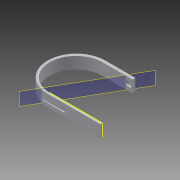
# Autodesk Inventor part: PinewoodFinish
Saved by Autodesk Inventor 2013 (Build 170138000, 138)
## iProperties
Created: 2015-05-15
Part Number: PinewoodFinish
Material: Generic
Document SubType Name: Modeling
Designer: joshgunnar
Density: 1 g/cm^3
Author: joshgunnar
Autodesk Inventor part; units mm, degrees
ref_plane "YZ Plane" through (0, 0, 0) normal (1, 0, 0) x (0, 1, 0)
ref_plane "XZ Plane" through (0, 0, 0) normal (0, 1, 0) x (-1, 0, 0)
sketch "Sketch1" plane through (0, 0, 0) normal (0, 0, 1) x (1, 0, 0)
  line L0 (0, 0) -> (88.9, 0)
  line L1 (88.9, 0) -> (88.9, 3.5)
  line L2 (88.9, 3.5) -> (0, 3.5)
  line L3 (0, 3.5) -> (0, 0)
  line L4 (0, 92.4) -> (50.8, 92.4)
  line L5 (50.8, 92.4) -> (50.8, 97.4)
  line L6 (50.8, 97.4) -> (0, 97.4)
  line L7 (0, 97.4) -> (0, 92.4)
  arc A0 (0, 92.4) -> (0, 3.5) centre (0, 47.95) ccw
  arc A1 (0, 97.4) -> (0, 0) centre (0, 48.7) ccw
  dimension "d0" = 88.9
  dimension "d1" = 3.5
  dimension "d2" = 50.8
  dimension "d3" = 5
  dimension "d4" = 88.9
  constraints: 16 end point, 4 parallel, 4 point on circle, 4 tangent, 2 centre point, 2 horizontal, 2 perpendicular
  measures "d0" distance of L2.end L1.end
  measures "d1" distance of L1.end L0.end
  measures "d2" distance of L6.end L5.end
  measures "d3" distance of L5.end L4.end
  measures "d4" distance between parallel lines of L2 L4
extrude "Extrusion1" add sketch "Sketch1" along normal blind 20
sketch "Sketch2" plane through (0, 3.5, 0) normal (0, 1, 0) x (1, 0, 0)
  line L0 (88.9, 0) -> (0, 0) projected
  line L1 (0, 0) -> (0, -20) projected
  line L2 (88.9, -20) -> (0, -20) projected
  line L3 (88.9, 0) -> (88.9, -20) projected
sketch "Sketch3" plane through (0, 92.4, 0) normal (0, -1, 0) x (1, 0, 0)
  line L0 (0, 0) -> (0, 20) projected
  line L1 (47.95, 6.5) -> (40.95, 6.5)
  line L2 (40.95, 6.5) -> (40.95, 13.5)
  line L3 (40.95, 13.5) -> (47.95, 13.5)
  line L4 (47.95, 13.5) -> (47.95, 6.5)
  line L5 (47.95, 6.5) -> (40.95, 13.5) construction
  line L6 (40.95, 6.5) -> (47.95, 13.5) construction
  point P0 (44.45, 10)
  dimension "d8" = 7
  dimension "d9" = 7
  dimension "d10" = 44.45
  constraints: 12 end point, 2 midpoint, 2 parallel, 1 horizontal, 1 perpendicular
  measures "d8" distance of L2.end L3.end
  measures "d9" distance of L1.end L2.end
  measures "d10" distance from line of L0 point (44.45, 10)
extrude "Extrusion2" cut sketch "Sketch3" against normal blind 3
ref_plane "Work Plane1" through (40.95, 95.4, 6.5) normal (-0.8660254, 0.5, 0) x (0, 0, 1)
sketch "Sketch4" plane through (40.95, 95.4, 6.5) normal (-0.8660254, 0.5, 0) x (0, 0, 1)
  line L0 (0, 0) -> (7, 0) projected
  line L1 (-6.5, -104.4399) -> (13.5, -104.4399) projected
  line L2 (13.5, -104.4399) -> (13.5, -108.0877) projected
  line L3 (13.5, -108.0877) -> (-6.5, -108.0877) projected
  line L4 (-6.5, -108.0877) -> (-6.5, -104.4399) projected
  line L5 (13.5, -3.4641) -> (-6.5, -3.4641) projected
  line L6 (-6.5, -3.4641) -> (-6.5, 2.3094) projected
  line L7 (-6.5, 2.3094) -> (13.5, 2.3094) projected
  line L8 (13.5, 2.3094) -> (13.5, -3.4641) projected
  line L9 (7, 0) -> (0, 0)
  line L10 (0, 0) -> (0, -3)
  line L11 (0, -3) -> (7, -3)
  line L12 (7, -3) -> (7, 0)
  point P0 (-6.5, -103.0938)
  dimension "d14" = 3
  constraints: 8 end point, 2 parallel, 1 horizontal, 1 perpendicular
  measures "d14" distance of L10.end L9.end
extrude "Extrusion3" cut sketch "Sketch4" along normal through all both and the other way through all contours L0 L12 L11 L10
sketch "Sketch5" plane through (0, 3.5, 0) normal (0, 1, 0) x (1, 0, 0)
  line L0 (0, 0) -> (0, -20) projected
  line L1 (47.95, -13.5) -> (40.95, -13.5)
  line L2 (40.95, -13.5) -> (40.95, -6.5)
  line L3 (40.95, -6.5) -> (47.95, -6.5)
  line L4 (47.95, -6.5) -> (47.95, -13.5)
  line L5 (47.95, -13.5) -> (40.95, -6.5) construction
  line L6 (40.95, -13.5) -> (47.95, -6.5) construction
  line L7 (38.45, -16) -> (50.45, -16)
  line L8 (50.45, -16) -> (50.45, -4)
  line L9 (50.45, -4) -> (38.45, -4)
  line L10 (38.45, -4) -> (38.45, -16)
  line L11 (38.45, -16) -> (50.45, -4) construction
  line L12 (50.45, -16) -> (38.45, -4) construction
  point P0 (44.45, -10)
  dimension "d17" = 7
  dimension "d18" = 7
  dimension "d19" = 44.45
  dimension "d20" = 12
  dimension "d21" = 12
  constraints: 24 end point, 4 midpoint, 4 parallel, 2 horizontal, 2 perpendicular
  measures "d17" distance of L2.end L3.end
  measures "d18" distance of L1.end L2.end
  measures "d19" distance from line of L0 point (44.45, -10)
  measures "d20" distance of L9.end L8.end
  measures "d21" distance of L8.end L7.end
extrude "Extrusion4" add sketch "Sketch5" along normal blind 3
ref_plane "Work Plane2" through (40.95, 3.5, 3.25) normal (-0.9659258, -0.258819, 0) x (0, 0, 1)
sketch "Sketch6" plane through (40.95, 3.5, 3.25) normal (-0.9659258, -0.258819, 0) x (0, 0, 1)
  line L0 (10.25, 0) -> (3.25, 0) projected
  line L1 (16.75, -3.6235) -> (-3.25, -3.6235) projected
  line L2 (-3.25, -3.6235) -> (-3.25, 0) projected
  line L3 (-3.25, 0) -> (0.75, 0) projected
  line L4 (0.75, 0) -> (0.75, 3.1058) projected
  line L5 (0.75, 3.1058) -> (12.75, 3.1058) projected
  line L6 (12.75, 3.1058) -> (12.75, 0) projected
  line L7 (12.75, 0) -> (16.75, 0) projected
  line L8 (16.75, 0) -> (16.75, -3.6235) projected
  line L9 (16.75, 92.0361) -> (-3.25, 92.0361) projected
  line L10 (-3.25, 92.0361) -> (-3.25, 97.2124) projected
  line L11 (-3.25, 97.2124) -> (16.75, 97.2124) projected
  line L12 (16.75, 97.2124) -> (16.75, 92.0361) projected
  line L13 (10.25, 0) -> (3.25, 0)
  line L14 (3.25, 0) -> (3.25, 3.1058)
  line L15 (3.25, 3.1058) -> (10.25, 3.1058)
  line L16 (10.25, 3.1058) -> (10.25, 0)
  point P0 (-3.25, 7.2179)
  constraints: 8 end point, 2 parallel, 1 horizontal, 1 perpendicular, 1 point on line
extrude "Extrusion5" cut sketch "Sketch6" along normal through all both and the other way through all contours L0 L14 L5 L16
sketch "Sketch7" plane through (0, 6.5, 0) normal (0, 1, 0) x (1, 0, 0)
  line L0 (40.1462, -13.5) -> (40.1462, -6.5) projected
  line L1 (38.45, -4) -> (38.45, -16) projected
  line L2 (38.45, -16) -> (38.45, -4) projected
  line L3 (38.45, -4) -> (50.45, -4) projected
  line L4 (50.45, -4) -> (50.45, -6.5) projected
  line L5 (50.45, -6.5) -> (40.1462, -6.5) projected
  line L6 (40.1462, -6.5) -> (40.1462, -13.5) projected
  line L7 (40.1462, -13.5) -> (50.45, -13.5) projected
  line L8 (50.45, -13.5) -> (50.45, -16) projected
  line L9 (50.45, -16) -> (38.45, -16) projected
  line L10 (-16.053, 0) -> (-16.053, -20) projected
  line L11 (-16.053, -20) -> (-24.3074, -20) projected
  line L12 (-24.3074, -20) -> (-24.3074, 0) projected
  line L13 (-24.3074, 0) -> (-16.053, 0) projected
  line L14 (40.1462, -13.5) -> (38.45, -13.5) projected
  line L15 (40.1462, -6.5) -> (38.45, -6.5) projected
  point P0 (0, 0)
extrude "Extrusion6" cut sketch "Sketch7" against normal blind 3 contours L14 L1 L15 L0
sketch "Sketch8" plane through (0, 0, 0) normal (0, -1, 0) x (1, 0, 0)
  line L0 (27.8878, 13.5) -> (27.8878, 6.5) projected
  line L1 (27.8878, 6.5) -> (15.8878, 6.5) projected
  line L2 (15.8878, 6.5) -> (15.8878, 13.5) projected
  line L3 (15.8878, 13.5) -> (27.8878, 13.5) projected
  line L4 (15.8878, 13.5) -> (-12.9863, 13.5)
  line L5 (-12.9863, 13.5) -> (-12.9863, 6.5)
  line L6 (-12.9863, 6.5) -> (15.8878, 6.5)
  line L7 (15.8878, 6.5) -> (15.8878, 13.5)
  constraints: 8 end point, 2 parallel, 1 horizontal, 1 perpendicular
extrude "Extrusion7" cut sketch "Sketch8" against normal blind 1.5
body "Solid1"
